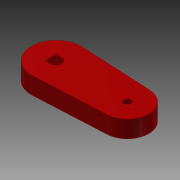
# Autodesk Inventor part: 20013
Saved by Autodesk Inventor 2014 (Build 180170000, 170)
## iProperties
Created: 2013-10-20
Part Number: 20013
Material: ABS Plastic
Document SubType Name: Modeling
Designer: Edward
Density: 1.06 g/cm^3
Appearance: Smooth - Red
Author: Edward
Autodesk Inventor part; units mm, degrees
ref_plane "YZ Plane" through (0, 0, 0) normal (1, 0, 0) x (0, 1, 0)
ref_plane "XZ Plane" through (0, 0, 0) normal (0, 1, 0) x (-1, 0, 0)
ref_plane "XY Plane" through (0, 0, 0) normal (0, 0, 1) x (1, 0, 0)
sketch "Sketch1" plane through (0, 0, 0) normal (0, 0, 1) x (1, 0, 0)
  circle A0 centre (0, 0) radius 4
  arc A1 (0, 17.5) -> (0, -17.5) centre (0, 0) ccw
  arc A2 (50.7435, -14.9816) -> (50.7435, 14.9816) centre (50, 0) ccw
  line L0 (0, 17.5) -> (50.7435, 14.9816)
  line L1 (50.7435, -14.9816) -> (0, -17.5)
  circle A3 centre (50, 0) radius 2.5
  point P0 (1.8995, -17.4057)
  point P1 (1.8995, 17.4057)
  dimension "d0" = 8
  dimension "d1" = 35
  dimension "d2" = 30
  dimension "d3" = 50
  dimension "d4" = 0
  dimension "d5" = 5
  constraints: 4 centre point, 4 end point, 4 point on circle, 3 coincident, 2 point on line, 2 tangent
  measures "d0" diameter of A0
  measures "d1" diameter of A1
  measures "d2" diameter of A2
  measures "d3" distance of A1.centre A2.centre
  measures "d4" vertical distance of point (0, 0) A2.centre
  measures "d5" diameter of A3
extrude "Extrusion1" add sketch "Sketch1" along normal blind 12
sketch "Sketch7" plane through (0, 0, 0) normal (0, 0, -1) x (-1, 0, 0)
  circle A0 centre (-50, 0) radius 2.5 projected
  arc A1 (-50.7435, 14.9816) -> (-50.7435, -14.9816) centre (-50, 0) ccw projected
  circle A2 centre (-50, 0) radius 8.25
  dimension "d23" = 16.5
  constraints: 1 centre point, 1 coincident
  measures "d23" diameter of A2
extrude "Extrusion7" cut sketch "Sketch7" against normal blind 6
sketch "Sketch8" plane through (0, 0, 12) normal (0, 0, 1) x (1, 0, 0)
  circle A0 centre (0, 0) radius 4 projected
  line L0 (-4, 4) -> (0, 4)
  line L1 (0, 4) -> (0, -4)
  line L2 (0, -4) -> (-4, -4)
  line L3 (-4, -4) -> (-4, 4)
  dimension "d26" = 8
  dimension "d27" = 4
  constraints: 8 end point, 2 parallel, 2 point on circle, 1 horizontal, 1 perpendicular
  measures "d26" distance between parallel lines of L2 L0
  measures "d27" distance of L0.start L0.end
extrude "Extrusion8" cut sketch "Sketch8" against normal through all contours L1 A0 | A0 L3 L0 | L2 L3 A0 picked at (-0.5785, -1.2013)
sketch "Sketch9" plane through (-4, -4, 12) normal (1, 0, 0) x (0, 0, -1)
  circle A0 centre (6, 4) radius 2.5
  point P0 (12, 4)
  dimension "d30" = 5
  constraints: 1 centre point
  measures "d30" diameter of A0
extrude "Extrusion9" cut sketch "Sketch9" against normal through all
sketch "Sketch10" plane through (-4, -4, 12) normal (1, 0, 0) x (0, 0, -1)
  circle A0 centre (6, 4) radius 2.5 projected
  line L0 (1.3812, 4) -> (3.6906, 8)
  line L1 (3.6906, 8) -> (8.3094, 8)
  line L2 (8.3094, 8) -> (10.6188, 4)
  line L3 (10.6188, 4) -> (8.3094, 0)
  line L4 (8.3094, 0) -> (3.6906, 0)
  line L5 (3.6906, 0) -> (1.3812, 4)
  point P0 (12, 4)
  dimension "d33" = 8
  constraints: 12 end point, 1 coincident, 13 other
  measures "d33" distance between parallel lines of L2 L5
extrude "Extrusion10" cut sketch "Sketch10" against normal blind 4.5
body "Solid1"
